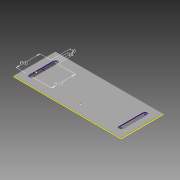
# Autodesk Inventor part: FelsoLemezVizhutes
Saved by Autodesk Inventor 2015 (Build 190159000, 159)
## iProperties
Created: 2014-10-31
Part Number: FelsoLemezVizhutes
Material: Steel, Alloy
Document SubType Name: Modeling
Designer: laca
Density: 7.73 g/cm^3
Appearance: Semi-Polished
Sheet Metal Rule: Default
Mass: 161.371 g
Surface Area: 427.644 cm^2
Volume: 20.8759 cm^3
Author: laca
Autodesk Inventor part; units mm, degrees
ref_plane "YZ Plane" through (0, 0, 0) normal (1, 0, 0) x (0, 1, 0)
ref_plane "XZ Plane" through (0, 0, 0) normal (0, 1, 0) x (-1, 0, 0)
ref_plane "XY Plane" through (0, 0, 0) normal (0, 0, 1) x (1, 0, 0)
derived "AlsoLemezVizhutesVer2.ipt"
sketch "Sketch1" plane through (0, 0, 0) normal (0, 1, 0) x (-1, 0, 0)
  circle A0 centre (7.2361, 13.6424) radius 1.5
  line L0 (0, 1.6974) -> (0, -1.2933)
  line L1 (1.3539, 0) -> (-1.1645, 0)
  circle A1 centre (7.2361, -39.3576) radius 1.5
  circle A2 centre (-92.7639, 13.6424) radius 1.5
  circle A3 centre (-92.7639, -39.3576) radius 1.5
  line L2 (17.2361, 33.6424) -> (-101.8474, 33.6424)
  line L3 (-101.8474, 33.6424) -> (-101.8474, -59.3576)
  line L4 (-101.8474, -59.3576) -> (17.2361, -59.3576)
  line L5 (17.2361, -59.3576) -> (17.2361, 33.6424)
  line L6 (-220.9309, 33.6424) -> (-101.8474, 33.6424)
  line L7 (-220.9309, -59.3576) -> (-220.9309, 33.6424)
  line L8 (-101.8474, -59.3576) -> (-220.9309, -59.3576)
  circle A4 centre (-210.9309, 13.6424) radius 1.5
  circle A5 centre (-210.9309, -39.3576) radius 1.5
  circle A6 centre (-110.9309, 13.6424) radius 1.5
  circle A7 centre (-110.9309, -39.3576) radius 1.5
  line L9 (-2.7639, -39.3576) -> (-2.7639, 13.6424) construction
  line L10 (2.2361, -39.3576) -> (2.2361, 13.6424)
  line L11 (-7.7639, 13.6424) -> (-7.7639, -39.3576)
  arc A8 (-7.7639, -39.3576) -> (2.2361, -39.3576) centre (-2.7639, -39.3576) ccw
  arc A9 (2.2361, 13.6424) -> (-7.7639, 13.6424) centre (-2.7639, 13.6424) ccw
  line L12 (-205.9309, -39.3576) -> (-205.9309, 13.6424)
  line L13 (-195.9309, 13.6424) -> (-195.9309, -39.3576)
  arc A10 (-205.9309, -39.3576) -> (-195.9309, -39.3576) centre (-200.9309, -39.3576) ccw
  arc A11 (-195.9309, 13.6424) -> (-205.9309, 13.6424) centre (-200.9309, 13.6424) ccw
  point P0 (0, 0)
  point P1 (-2.7639, -12.8576)
  dimension "d102" = 53
  dimension "d103" = 53
  dimension "d104" = 10
  dimension "d105" = 10
  measures "d102" distance of A0.centre A1.centre
  measures "d103" distance of L9.end L9.start
  measures "d104" distance between parallel lines of L11 L10
  measures "d105" distance from line of L9 A1.centre
extrude "Extrusion4" add sketch "Sketch1" along normal blind 1 contours L5 L4 L3 L2 | L3 L8 L7 L6 | A8 L11 A9 L10 | L12 A11 L13 A10
extrude "Extrusion5" cut sketch "Sketch1" along normal blind 10 contours A8 L11 A9 L10 | L12 A11 L13 A10
equation "\"d103\" = d102"
equation "\"BendRadius\" = Thickness"
equation "\"BendReliefWidth\" = Thickness"
equation "\"BendReliefDepth\" = 0.5 * Thickness"
equation "\"CornerReliefSize\" = 4 * Thickness"
equation "\"MinimumRemnant\" = 2 * Thickness"
equation "\"TransitionRadius\" = BendRadius"
equation "\"JacobiRadiusSize\" = Thickness"
equation "\"GapSize\" = Thickness"
equation "\"Thickness\" = 0.5"
body "Solid3"
